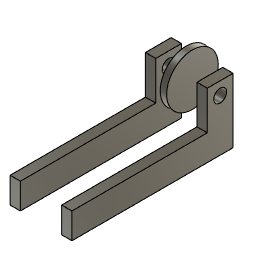
200405_jointExample_disk&LBars_v2 (Autodesk Fusion 360 design; units mm, degrees)
Autodesk Fusion 360 part; units mm, degrees
sketch "Sketch1" plane through (0, 0, 0) normal (1, 0, 0) x (0, 1, 0) in component "L-bar"
  line L0 (0, 0) -> (125, 0)
  line L1 (125, 0) -> (125, 20)
  line L2 (125, 20) -> (0, 20)
  line L3 (0, 20) -> (0, 0)
  line L4 (125, 20) -> (105, 20)
  line L5 (105, 20) -> (105, 50)
  line L6 (105, 50) -> (125, 50)
  line L7 (125, 50) -> (125, 20)
  circle A0 centre (115, 40) radius 5
  constraint horizontal L0
  constraint vertical L1
  constraint horizontal L2
  constraint vertical L3
  constraint coincident L0.start L3.end
  constraint horizontal L4
  constraint vertical L5
  constraint horizontal L6
  constraint vertical L7
extrude "Extrude1" add sketch "Sketch1" along normal blind 8 makes body 1 in component "L-bar"
sketch "Sketch1 (2)" plane through (8, 0, 0) normal (1, 0, 0) x (0, 1, 0) in component "disk"
  circle A0 centre (115, 40) radius 5
  line L0 (105, 20) -> (0, 20)
  line L1 (0, 20) -> (0, 0)
  line L2 (0, 0) -> (125, 0)
  line L3 (125, 0) -> (125, 50)
  line L4 (125, 50) -> (105, 50)
  line L5 (105, 50) -> (105, 20)
  circle A1 centre (25, 75) radius 20
extrude "Extrude1'" add sketch "Sketch1 (2)" along normal blind 5 separate body contours A1 makes body 2 in component "disk"
component "L-bar" placed x (1, 0, 0) y (0, 1, 0) z (0, 0, 1) at (0, 0, 0)
component "L-bar" placed x (1, 0, 0) y (0, 1, 0) z (0, 0, 1) at (-40, 0, 0)
component "disk" placed x (1, 0, 0) y (0, 1, 0) z (0, 0, 1) at (-26.5, 90, -35)
